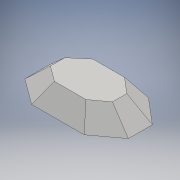
# Autodesk Inventor part: Cover end
Saved by Autodesk Inventor 2016 (Build 200138000, 138)
## iProperties
Created: 2017-08-22
Part Number: Cover end
Material: Generic
Document SubType Name: Modeling
Designer: m227586
Density: 1 g/cm^3
Appearance: Default
Author: m227586
Autodesk Inventor part; units mm, degrees
ref_plane "YZ Plane" through (0, 0, 0) normal (1, 0, 0) x (0, 1, 0)
ref_plane "XZ Plane" through (0, 0, 0) normal (0, 1, 0) x (-1, 0, 0)
sketch "Sketch2" plane through (0, 0, 0) normal (0, 0, 1) x (1, 0, 0)
  line L0 (7.8638, 351.0024) -> (-267.6362, 351.0024)
  line L1 (-267.6362, 351.0024) -> (-534, 125.5)
  line L2 (-534, 125.5) -> (-534, -125.5)
  line L3 (-534, -125.5) -> (-267.6362, -321.9976)
  line L4 (-267.6362, -321.9976) -> (7.8638, -321.9976)
  line L5 (7.8638, 351.0024) -> (7.8638, -321.9976) construction
  line L6 (-534, 0) -> (0, 0) construction
  line L7 (7.8638, 351.0024) -> (283.3638, 351.0024)
  line L8 (283.3638, 351.0024) -> (549.7276, 125.5)
  line L9 (549.7276, 125.5) -> (549.7276, -125.5)
  line L10 (549.7276, -125.5) -> (283.3638, -321.9976)
  line L11 (283.3638, -321.9976) -> (7.8638, -321.9976)
  dimension "d19" = 673
  dimension "d20" = 275.5
  dimension "d21" = 251
  dimension "d22" = 349
  dimension "d23" = 331
  dimension "d24" = 275.5
  dimension "d25" = 534
  constraints: 24 end point, 4 symmetric about line, 2 perpendicular, 2 vertical, 1 horizontal, 1 horizontal alignment, 1 midpoint
  measures "d19" distance of L0.start L4.end
  measures "d20" distance of L0.start L0.end
  measures "d21" distance of L1.end L2.end
  measures "d22" distance of L0.end L1.end
  measures "d23" distance of L2.end L3.end
  measures "d24" distance of L3.end L4.end
  measures "d25" distance of L6.start L6.end
ref_plane "Work Plane1" through (0, 0, 200) normal (0, 0, 1) x (1, 0, 0)
sketch "Sketch3" plane through (0, 0, 200) normal (0, 0, 1) x (1, 0, 0)
  line L0 (7.8638, 210.6014) -> (-157.4362, 210.6014)
  line L1 (-157.4362, 210.6014) -> (-317.2545, 75.3)
  line L2 (-317.2545, 75.3) -> (-317.2545, -75.3)
  line L3 (-317.2545, -75.3) -> (-157.4362, -193.1986)
  line L4 (-157.4362, -193.1986) -> (7.8638, -193.1986)
  line L5 (7.8638, 210.6014) -> (173.1638, 210.6014)
  line L6 (173.1638, 210.6014) -> (332.9821, 75.3)
  line L7 (332.9821, 75.3) -> (332.9821, -75.3)
  line L8 (332.9821, -75.3) -> (173.1638, -193.1986)
  line L9 (173.1638, -193.1986) -> (7.8638, -193.1986)
  point P0 (0, 0)
  point P1 (0, 0)
  point P2 (0, 0)
  point P3 (0, -225.5024)
  point P4 (7.8638, 125.5)
  point P5 (7.8638, 0)
  point P6 (7.8638, -85.1014)
  dimension "d34" = 165.3
  dimension "d35" = 150.6
  dimension "d36" = 209.4
  dimension "d37" = 198.6
  dimension "d38" = 165.3
  constraints: 20 end point, 1 coincident, 1 horizontal, 1 perpendicular, 1 vertical
  measures "d34" distance of L0.start L0.end
  measures "d35" distance of L1.end L2.end
  measures "d36" distance of L0.end L1.end
  measures "d37" distance of L2.end L4.start
  measures "d38" distance of L4.start L4.end
loft "Loft1" add profiles "Sketch2", "Sketch3"
shell "Shell1" thickness 3 removed faces 1 at (191.5305, -97.6643, 0)
body "Solid1"
